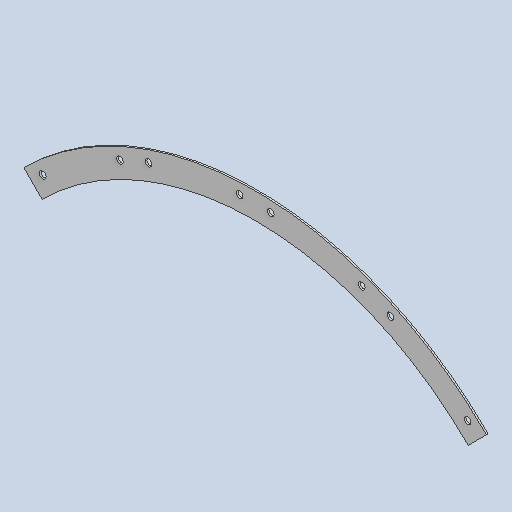
# Autodesk Inventor part: DMF2.0 01 43 Gear rim 3
Saved by Autodesk Inventor 2025 (Build 290162010, 162A)
## iProperties
Created: 2024-04-30
Part Number: DMF2.0 01 43 Gear rim 3
Material: Generic
Document SubType Name: Sheet Metal
Designer: admin
Stock Number: Барабан_Сектор_Усилителя
Density: 1 g/cm^3
Sheet Metal Rule: Default
Sheet Metal Width: 0,000 mm
Sheet Metal Length: 0,000 mm
Sheet Metal Area: 0,000 mm^2
Appearance: Default
Author: pokla
Autodesk Inventor part; units mm, degrees
ref_plane "YZ Plane" through (0, 0, 0) normal (1, 0, 0) x (0, 1, 0)
ref_plane "XZ Plane" through (0, 0, 0) normal (0, 1, 0) x (-1, 0, 0)
ref_plane "XY Plane" through (0, 0, 0) normal (0, 0, 1) x (1, 0, 0)
sketch "Sketch1" plane through (0, 0, 0) normal (0, 0, 1) x (1, 0, 0)
  circle A0 centre (0, 0) radius 350
  circle A1 centre (0, 0) radius 380
  line L0 (0, 0) -> (-268.7006, 268.7006)
  line L1 (0, 0) -> (0, 380)
  line L2 (0, 0) -> (268.7006, 268.7006)
  point P0 (-247.4874, 247.4874)
  point P1 (247.4874, 247.4874)
  dimension "d30" = 90
  dimension "d31" = 760
  dimension "d32" = 700
  measures "d30" angle of L2 L0
  measures "d31" diameter of A1
  measures "d32" diameter of A0
extrude "Plate1" add sketch "Sketch1" against normal blind 2 contours A0 L1 A1 L2 | L0 A1 L1 A0
sketch "Sketch2" plane through (0, 0, 0) normal (0, 0, 1) x (1, 0, 0)
  circle A0 centre (0, 0) radius 367.5
  arc A1 (268.7006, 268.7006) -> (-268.7006, 268.7006) centre (0, 0) ccw projected
  line L0 (0, 0) -> (268.7006, 268.7006) construction
  line L1 (0, 0) -> (246.7979, 272.2995) construction
  line L2 (157.1265, 332.2161) -> (0, 0) construction
  line L3 (0, 0) -> (0, 367.5) construction
  line L4 (0, 0) -> (18.0324, 367.0573) construction
  line L5 (0, 0) -> (123.807, 346.0174) construction
  dimension "d34" = 735
  dimension "d35" = 2.812
  dimension "d36" = 16.875
  dimension "d44" = 2.812
  dimension "d45" = 16.875
  constraints: 12 end point, 5 point on circle, 1 centre point, 1 coincident, 1 vertical
  measures "d34" diameter of A0
  measures "d35" angle of L0 L1
  measures "d36" angle of L1 L2
  measures "d44" angle of L4 L3
  measures "d45" angle of L5 L4
hole "Hole1" at (246.7979, 272.2995, 0) at (157.1265, 332.2161, 0) at (123.807, 346.0174, 0) at (18.0324, 367.0573, 0) direction (0, 0, -1) diameter 8 end through all
pattern_circular "Circular Pattern1" count 2 over 45 about axis through (0, 0, -10) along (0, 0, 1) of "Hole1"
equation "\"d31\" = Колесо_диам_1"
equation "\"d32\" = Колесо_диам_2"
equation "\"d44\" = d35"
equation "\"d45\" = d36"
equation "\"d42\" = Thickness"
equation "\"d15\" = Thickness"
equation "\"BendRadius\" = Thickness"
equation "\"BendReliefWidth\" = Thickness"
equation "\"BendReliefDepth\" = 0.5 * Thickness"
equation "\"CornerReliefSize\" = 4 * Thickness"
equation "\"MinimumRemnant\" = 2 * Thickness"
equation "\"TransitionRadius\" = BendRadius"
equation "\"JacobiRadiusSize\" = BendRadius"
equation "\"GapSize\" = Thickness"
equation "\"Колесо_диам_1\" = 760"
equation "\"Колесо_диам_2\" = 700"
equation "\"Thickness\" = 2"
body "Solid1"
